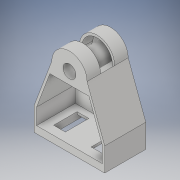
# Autodesk Inventor part: LampeSolaire2_LedAmoviblePart 3D printed
Saved by Autodesk Inventor 2019 (Build 230136000, 136)
## iProperties
Created: 2020-09-24
Part Number: LampeSolaire2_LedAmoviblePart 3D printed
Material: Generic
Document SubType Name: Modeling
Designer: nicolas
Density: 1 g/cm^3
Appearance: Default
Author: nicolas
## iProperties of the stored document LampeSolaire2_LedAmoviblePart_3DPrint.ipt
Created: 2020-10-22
Part Number: LampeSolaire2_LedAmoviblePart_3DPrint
Material: Generic
Document SubType Name: Modeling
Designer: nicolas
Density: 1 g/cm^3
Appearance: Default
Author: nicolas
Autodesk Inventor part; units mm, degrees
note: some values were not read from the file. Chosen so that the rebuilt part matches the saved one: direction of "Hole3".
ref_plane "YZ Plane" through (0, 0, 0) normal (1, 0, 0) x (0, 1, 0)
sketch "Sketch1" plane through (0, 0, 0) normal (0, 0, 1) x (1, 0, 0)
  arc A0 (7.5, 0) -> (-7.5, 0) centre (0, 0) ccw
  line L0 (-7.5, 0) -> (-15, -20)
  line L1 (7.5, 0) -> (15, -20)
  line L2 (-7.5, 0) -> (7.5, 0) construction
  line L3 (-15, -30) -> (15, -30)
  line L4 (-15, -30) -> (15, -30) construction
  circle A1 centre (0, 0) radius 2.75
  line L5 (-15, -20) -> (-15, -30)
  line L6 (15, -20) -> (15, -30)
  dimension "d0" = 15
  dimension "d8" = 5.5
  dimension "d67" = 30
  dimension "d68" = 30
  dimension "d96" = 10
  constraints: 14 end point, 2 centre point, 2 coincident, 2 equal length, 2 horizontal, 2 point on circle, 2 vertical, 1 midpoint
  measures "d0" diameter of A0
  measures "d8" diameter of A1
  measures "d67" distance from line of point (0, 0) L3
  measures "d68" distance of L3.start L3.end
  measures "d96" distance of L0.end L3.start
extrude "Extrusion1" add sketch "Sketch1" along normal blind 17.5
shell "Shell2" thickness 1 removed faces 1 at (0.1105, -14.2433, 17.5)
thicken "Thicken5" operation add thickness 2 both sides no extend neighbours no toward (0, 1, 0) faces at (-4.6667, -29, 6.5)
sketch "Sketch12" plane through (-15, -30, 0) normal (0, -1, 0) x (1, 0, 0)
  line L0 (0, 0) -> (30, 0) projected
  line L1 (30, 0) -> (30, 17.5) projected
  line L2 (0, 17.5) -> (30, 17.5) projected
  line L3 (0, 0) -> (0, 17.5) projected
  line L4 (25.5, 16.25) -> (4.5, 16.25)
  line L5 (4.5, 16.25) -> (4.5, 1.25)
  line L6 (4.5, 1.25) -> (25.5, 1.25)
  line L7 (25.5, 1.25) -> (25.5, 16.25)
  line L8 (25.5, 16.25) -> (25.5, 17.5)
  line L9 (21.4976, 17.5) -> (29, 17.5) projected
  line L10 (25.5, 1.25) -> (25.5, 0)
  line L11 (0, 0) -> (30, 0) projected
  point P0 (15, 0)
  dimension "d74" = 21
  dimension "d75" = 15
  dimension "d77" = 4.5
  dimension "d78" = 4.5
  dimension "d79" = 1.25
  constraints: 12 end point, 3 perpendicular, 2 parallel, 2 point on line, 1 collinear, 1 horizontal
  measures "d74" distance of L6.end L5.end
  measures "d75" distance of L5.end L4.end
  measures "d77" distance between parallel lines of L1 L7
  measures "d78" distance between parallel lines of L3 L5
  measures "d79" distance between parallel lines of L0 L6
extrude "Extrusion6" cut sketch "Sketch12" against normal blind 2 contours L6 L5 L4 L7
sketch "Sketch13" plane through (-15, -28, 0) normal (0, -1, 0) x (1, 0, 0)
  line L0 (25.5, 16.25) -> (25.5, 1.25) projected
  line L1 (4.5, 1.25) -> (4.5, 16.25) projected
  line L2 (4.5, 13.75) -> (9.5, 13.75)
  line L3 (9.5, 13.75) -> (9.5, 3.75)
  line L4 (9.5, 3.75) -> (4.5, 3.75)
  line L5 (4.5, 3.75) -> (4.5, 13.75)
  line L6 (4.5, 16.25) -> (25.5, 16.25) projected
  line L7 (25.5, 1.25) -> (4.5, 1.25) projected
  line L8 (25.5, 13.75) -> (20.5, 13.75)
  line L9 (20.5, 13.75) -> (20.5, 3.75)
  line L10 (20.5, 3.75) -> (25.5, 3.75)
  line L11 (25.5, 3.75) -> (25.5, 13.75)
  point P0 (15, 0)
  dimension "d82" = 5
  dimension "d83" = 10
  dimension "d84" = 2.5
  dimension "d85" = 2.5
  dimension "d86" = 5
  dimension "d87" = 10
  dimension "d88" = 2.5
  dimension "d89" = 2.5
  constraints: 16 end point, 4 parallel, 2 horizontal, 2 perpendicular, 2 point on line
  measures "d82" distance of L3.end L4.end
  measures "d83" distance of L2.end L3.end
  measures "d84" distance between parallel lines of L6 L2
  measures "d85" distance between parallel lines of L7 L4
  measures "d86" distance of L10.end L9.end
  measures "d87" distance of L9.end L8.end
  measures "d88" distance between parallel lines of L6 L8
  measures "d89" distance between parallel lines of L7 L10
extrude "Extrusion7" cut sketch "Sketch13" against normal up to next contours L0 L10 L9 L8 | L2 L3 L4 L1
sketch "Sketch14" plane through (-15, -28, 0) normal (0, -1, 0) x (1, 0, 0)
  line L0 (4.5, 16.25) -> (25.5, 16.25) projected
  line L1 (25.5, 16.25) -> (25.5, 1.25) projected
  line L2 (4.5, 1.25) -> (4.5, 16.25) projected
  line L3 (25.5, 1.25) -> (4.5, 1.25) projected
  line L4 (15, 1.25) -> (15, 16.25) construction
  line L5 (25.5, 8.75) -> (4.5, 8.75) construction
  line L6 (4.5, 13.75) -> (4.5, 3.75) projected
  point P0 (15, 0)
  point P1 (15, 9.5)
  constraints: 4 end point, 4 midpoint
ref_plane "Work Plane2" through (0, -7.5, 0) normal (0, 1, 0) x (-1, 0, 0)
sketch "Sketch16" plane through (0, 0, 1) normal (0, 0, 1) x (1, 0, 0)
  line L0 (14, -27) -> (-14, -27) projected
  line L1 (0, -27) -> (0, -16.6699) construction
  point P0 (0, 0)
  point P1 (0, -22)
  point P2 (-0.2812, -15.3392)
  point P3 (3.9903, -15.1005)
  dimension "d97" = 5
  constraints: 2 end point, 1 midpoint, 1 point on line, 1 vertical
  measures "d97" distance from line of L0 point (0, -22)
hole "Hole3" at (0, -22, 1) direction (0, 0, -1) diameter 3.4 depth 1 clearance for "Hex Head Cap Screw ISO 24017" size "M3" standard "ISO"
sketch "Sketch17" plane through (0, 0, 1) normal (0, 0, 1) x (1, 0, 0)
  circle A0 centre (0, -22) radius 1.7 projected
  circle A1 centre (0, -22) radius 4.75
  point P0 (0, 0)
  dimension "d105" = 9.5
  constraints: 1 centre point, 1 coincident
  measures "d105" diameter of A1
extrude "Extrusion9" add sketch "Sketch17" along normal blind 2
sketch "Sketch18" plane through (0, 0, 0) normal (0, 0, -1) x (-1, 0, 0)
  circle A0 centre (0, -22) radius 1.7 projected
  circle A1 centre (0, -22) radius 2.75 construction
  line L0 (2.75, -20.4123) -> (2.75, -23.5877)
  line L1 (2.75, -23.5877) -> (0, -25.1754)
  line L2 (0, -25.1754) -> (-2.75, -23.5877)
  line L3 (-2.75, -23.5877) -> (-2.75, -20.4123)
  line L4 (-2.75, -20.4123) -> (0, -18.8246)
  line L5 (0, -18.8246) -> (2.75, -20.4123)
  point P0 (0, 0)
  dimension "d108" = 5.5
  constraints: 12 end point, 2 coincident, 1 centre point, 1 tangent, 1 vertical, 13 other
  measures "d108" diameter of A1
extrude "Extrusion10" cut sketch "Sketch18" against normal blind 2
ref_plane "Work Plane3" through (0, 7.5, 0) normal (0, 1, 0) x (-1, 0, 0)
sketch "Sketch19" plane through (0, 7.5, 0) normal (0, 1, 0) x (-1, 0, 0)
  line L0 (-14, 17.5) -> (14, 17.5) projected
  line L1 (0, 17.5) -> (0, 0) construction
  line L2 (-7.5, 11.75) -> (7.5, 11.75)
  line L3 (7.5, 11.75) -> (7.5, 5.75)
  line L4 (7.5, 5.75) -> (-7.5, 5.75)
  line L5 (-7.5, 5.75) -> (-7.5, 11.75)
  line L6 (-7.5, 11.75) -> (7.5, 5.75) construction
  line L7 (7.5, 11.75) -> (-7.5, 5.75) construction
  point P0 (0, 8.75)
  dimension "d111" = 15
  dimension "d112" = 6
  constraints: 14 end point, 4 midpoint, 2 parallel, 1 horizontal, 1 perpendicular, 1 vertical
  measures "d111" distance of L3.end L4.end
  measures "d112" distance of L2.end L3.end
extrude "Extrusion11" cut sketch "Sketch19" against normal up to next
sketch "Sketch22" plane through (0, 0, 17.5) normal (0, 0, 1) x (1, 0, 0)
  line L0 (-8.307, -5) -> (8.307, -5)
  line L1 (6.4976, -0.175) -> (14, -20.1813) projected
  line L2 (-14, -20.1813) -> (-6.4976, -0.175) projected
  arc A0 (6.4976, -0.175) -> (-6.4976, -0.175) centre (0, 0) ccw projected
  circle A1 centre (0, 0) radius 2.75 projected
  dimension "d117" = 5
  constraints: 2 end point, 2 point on line, 1 horizontal
  measures "d117" distance from line of point (0, 0) L0
extrude "Extrusion13" add sketch "Sketch22" against normal blind 2
body "Solid1"
